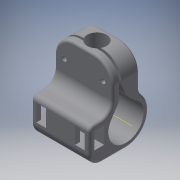
# Autodesk Inventor part: my_Sliding_Block_Complete
Saved by Autodesk Inventor 2016 (Build 200138000, 138)
## iProperties
Created: 2015-07-08
Part Number: my_Sliding_Block_Complete
Material: Generic
Document SubType Name: Modeling
Designer: Mathias L. Kjeldgaard
Density: 1 g/cm^3
Appearance: Default
Author: Mathias L. Kjeldgaard
Autodesk Inventor part; units mm, degrees
ref_plane "YZ Plane" through (0, 0, 0) normal (1, 0, 0) x (0, 1, 0)
sketch "Sketch1" plane through (0, 0, 0) normal (1, 0, 0) x (0, 1, 0)
  circle A0 centre (6.9957, 0) radius 7.5 construction
  circle A1 centre (6.9957, 0) radius 7.3
  line L0 (6.9957, -9.3) -> (-3.0043, -9.3)
  arc A2 (6.9957, -9.3) -> (13.8244, 6.3134) centre (6.9957, 0) ccw
  arc A3 (-8.0043, -4.3) -> (-3.0043, -9.3) centre (-3.0043, -4.3) ccw
  line L1 (6.9957, 0) -> (6.9957, 23.3) construction
  line L2 (12.4957, 4.8) -> (12.4957, 5.099)
  line L3 (12.4957, 9.7077) -> (12.4957, 23.3)
  arc A4 (12.4957, 9.7077) -> (13.8244, 6.3134) centre (17.4957, 9.7077) ccw
  line L4 (12.4957, 23.3) -> (5.0957, 23.3)
  line L5 (6.9957, 9.3) -> (5.0957, 9.3) construction
  line L6 (5.0957, 23.3) -> (5.0957, 16.4842)
  line L7 (12.4957, 9.7077) -> (12.4957, 4.8) construction
  line L8 (11.4281, 5.9069) -> (10.4435, 6.4345)
  arc A5 (5.0957, 16.4842) -> (11.4281, 5.9069) centre (17.0957, 16.4842) ccw
  line L9 (4.0957, 23.3) -> (1.4957, 23.3)
  line L10 (4.0957, 23.3) -> (4.0957, 10.3433)
  line L11 (1.4957, 23.3) -> (1.4957, 10.5)
  line L12 (-8.0043, 3.5) -> (-8.0043, -3.5)
  line L13 (-8.0043, -3.5) -> (-8.0043, -4.3)
  line L14 (-8.0043, 3.5) -> (-8.0043, 3.5)
  line L15 (-6.0043, 5.5) -> (-3.5043, 5.5)
  arc A6 (-3.5043, 5.5) -> (1.4957, 10.5) centre (-3.5043, 10.5) ccw
  line L16 (3.2629, 7.5803) -> (0.9116, 4.0341)
  arc A7 (3.2629, 7.5803) -> (4.0957, 10.3433) centre (-0.9043, 10.3433) ccw
  arc A8 (-6.0043, 5.5) -> (-8.0043, 3.5) centre (-6.0043, 3.5) ccw
  point P0 (0, 0)
  point P1 (12.4957, 7.4993)
  point P2 (6.9957, 7.3)
  point P3 (4.0957, 8.8363)
  point P4 (-8.0043, 5.5)
  dimension "d0" = 0.2
  dimension "d2" = 2
  dimension "d4" = 5
  dimension "d8" = 5
  dimension "d9" = 11
  dimension "d11" = 14
  dimension "d12" = 3.8
  dimension "d18" = 12
  dimension "d29" = 11
  dimension "d30" = 1
  dimension "d31" = 0
  dimension "d36" = 7
  dimension "d38" = 2
  dimension "d39" = 5
  dimension "d40" = 5
  dimension "d41" = 2
  dimension "d42" = 15
  dimension "d44" = 13
  constraints: 34 end point, 20 point on circle, 17 tangent, 11 point on line, 8 centre point, 6 perpendicular, 3 coincident, 3 parallel, 2 collinear, 1 horizontal, 2 other
  measures "d2" radial gap between concentric circles of A2 A1
  measures "d4" radius of A3
  measures "d8" radius of A4
  measures "d9" diameter of L3 L1
  measures "d11" distance from line of L5.start L4
  measures "d12" diameter of L6 L1
  measures "d18" radius of A5
  measures "d29" diameter of L11 L1
  measures "d30" distance between parallel lines of L6 L10
  measures "d31" distance from line of L1.end L9
  measures "d36" distance of L12.start L12.end
  measures "d38" distance of L12.start point (-8.004, 5.5)
  measures "d39" radius of A6
  measures "d40" radius of A7
  measures "d41" radius of A8
  measures "d42" distance from line of point (6.996, 0) L12
  measures "d44" horizontal distance of point (6.996, 0) A8.centre
ref_plane "Work Plane1" through (9.8693, -0.2503, -7.246) normal (1, 0, 0) x (0, 1, 0)
ref_plane "Work Plane2" through (-14.1307, -0.2503, -7.246) normal (-1, 0, 0) x (0, 0, 1)
extrude "Main body" add sketch "Sketch1" against normal up to surface (24 mm away) from surface at 9.8693 contours A1 L8 A5 L6 L4 L3 A4 A2 L0 A3 L13 L12 A8 L15 A6 L11 L9 L10 A7 L16
sketch "Sketch3" plane through (-14.1307, 5.0957, 23.3) normal (0, 0, 1) x (1, 0, 0)
  line L0 (24, 9.146) -> (24, -5.346) construction
  line L1 (0, -4.45) -> (0, 8.25) construction
  line L2 (0, -5.346) -> (0, 9.146) construction
  line L3 (0, 1.9) -> (24, 1.9) construction
  circle A0 centre (12, 1.9) radius 4
  point P0 (14.1307, -5.0957)
  dimension "d26" = 8
  constraints: 3 midpoint, 2 end point, 1 centre point
  measures "d26" diameter of A0
extrude "8mm hul" cut sketch "Sketch3" against normal blind 18.25
sketch "Sketch4" plane through (-14.1307, 1.4957, 10.5) normal (0, -1, 0) x (1, 0, 0)
  line L0 (0, 12.8) -> (0, 0) construction
  line L1 (0, 0) -> (24, 0) construction
  line L2 (24, 0) -> (24, 12.8) construction
  line L3 (0, 12.8) -> (24, 12.8) construction
  line L4 (8, 12.8) -> (16, 12.8) construction
  line L5 (9.245, 12.8) -> (14.755, 12.8) construction
  line L6 (8.4801, 12.8) -> (8.4801, 0) construction
  line L7 (15.5199, 12.8) -> (15.5199, 0) construction
  line L8 (15.5199, 12.8) -> (8.4801, 0) construction
  line L9 (12, 6.4) -> (12, 12.8) construction
  line L10 (8, 12.8) -> (8, 0) construction
  line L11 (16, 12.8) -> (16, 0) construction
  circle A0 centre (4, 5) radius 1
  circle A1 centre (20, 5) radius 1
  line L12 (20, 5) -> (4, 5) construction
  point P0 (14.1307, -10.5)
  dimension "d45" = 4
  dimension "d46" = 4
  dimension "d47" = 2
  dimension "d48" = 2
  dimension "d49" = 4
  dimension "d50" = 4
  dimension "d51" = 4
  dimension "d54" = 5
  constraints: 14 end point, 4 perpendicular, 4 point on line, 2 centre point, 2 midpoint, 1 parallel, 3 other
  measures "d45" distance between parallel lines of L9 L10
  measures "d46" distance between parallel lines of L11 L9
  measures "d47" diameter of A0
  measures "d48" diameter of A1
  measures "d49" distance from line of L2 L12.start
  measures "d50" distance from line of L0 L12.end
  measures "d51" distance from line of L11 L12.start
  measures "d54" distance between parallel lines of L1 L12
extrude "4mm Fastspændingshuller" cut sketch "Sketch4" against normal blind 10.25
sketch "Sketch5" plane through (-14.1307, 1.4957, 10.5) normal (0, -1, 0) x (1, 0, 0)
  line L0 (0, 12.8) -> (0, 0) construction
  line L1 (24, 0) -> (24, 12.8) construction
  line L2 (0, 12.8) -> (24, 12.8) construction
  line L3 (0, 4.8) -> (0, 0)
  line L4 (24, 0) -> (24, 4.8)
  line L5 (16, 12.8) -> (8, 12.8)
  arc A0 (8, 12.8) -> (0, 4.8) centre (8, 4.8) ccw
  arc A1 (24, 4.8) -> (16, 12.8) centre (16, 4.8) ccw
  line L6 (24, 0) -> (24, 4.8)
  line L7 (8, 12.8) -> (0, 12.8)
  line L8 (0, 12.8) -> (0, 4.8)
  line L9 (24, 12.8) -> (24, 4.8)
  line L10 (24, 12.8) -> (16, 12.8)
  point P0 (14.1307, -10.5)
  dimension "d57" = 8
  constraints: 16 end point, 7 tangent, 6 collinear, 5 point on circle, 5 point on line, 2 centre point, 1 equal radius, 1 perpendicular
  measures "d57" radius of A0
extrude "Afrunding v/ 8mm stang" cut sketch "Sketch5" against normal up to surface (11 mm away)
sketch "Sketch6" plane through (-14.1307, -3.0043, -9.3) normal (-1, 0, 0) x (0, 0, 1)
  arc A0 (15.6134, 16.8287) -> (0, 10) centre (9.3, 10) ccw construction
  line L0 (5.8, 1) -> (12.8, 1)
  line L1 (12.8, 1) -> (12.8, -3)
  line L2 (12.8, -3) -> (5.8, -3)
  line L3 (5.8, -3) -> (5.8, 1)
  point P0 (9.3, 3.0043)
  dimension "d60" = 7
  dimension "d61" = 4
  dimension "d62" = 9
  dimension "d63" = 3.5
  dimension "d64" = 3.5
  constraints: 8 end point, 2 parallel, 1 horizontal, 1 perpendicular
  measures "d60" distance between parallel lines of L3 L1
  measures "d61" distance between parallel lines of L0 L2
  measures "d62" distance from line of A0.centre L0
  measures "d63" distance from line of A0.centre L1
  measures "d64" distance from line of A0.centre L3
extrude "GT2 Belte hul Stort" cut sketch "Sketch6" against normal up to surface (24 mm away)
sketch "Sketch7" plane through (-14.1307, -8.0043, -4.3) normal (0, -1, 0) x (1, 0, 0)
  line L0 (0, 7.8) -> (0, 0) construction
  line L1 (24, 0.8) -> (24, 7.8) construction
  line L2 (0, 0.8) -> (24, 0.8) construction
  line L3 (0, 7.8) -> (0, 0.8) construction
  line L4 (0, 7.8) -> (24, 7.8) construction
  line L5 (2, 7.8) -> (6, 7.8)
  line L6 (6, 7.8) -> (6, 0.8)
  line L7 (6, 0.8) -> (2, 0.8)
  line L8 (2, 0.8) -> (2, 7.8)
  line L9 (18, 7.8) -> (22, 7.8)
  line L10 (22, 7.8) -> (22, 0.8)
  line L11 (22, 0.8) -> (18, 0.8)
  line L12 (18, 0.8) -> (18, 7.8)
  point P0 (14.1307, 4.3)
  dimension "d67" = 2
  dimension "d68" = 4
  dimension "d69" = 2
  dimension "d70" = 4
  constraints: 16 end point, 4 parallel, 4 point on line, 2 horizontal, 2 perpendicular
  measures "d67" distance between parallel lines of L8 L0
  measures "d68" distance between parallel lines of L6 L8
  measures "d69" distance between parallel lines of L1 L10
  measures "d70" distance between parallel lines of L12 L10
extrude "GT2 belte hul Lille" cut sketch "Sketch7" against normal blind 4.25
fillet "Ydre fillet" radius 1 16 edges at (9.8693, 1.9957, -9.3) (9.8693, -6.5398, -7.8355) (9.8693, -8.0043, -0.4) (9.8693, -7.4185, 4.9142) (9.8693, -4.7543, 5.5) (9.8693, 0.0313, 6.9645) (9.8693, 1.4957, 12.9) (7.5262, 1.4957, 20.9569) (-2.1307, 1.4957, 23.3) (-11.7875, 1.4957, 20.9569) (9.8693, 15.5164, -3.7266) (9.8693, 12.8397, 7.8852) (9.8693, 12.4957, 12.5039) (-11.7875, 12.4957, 20.9569) (-2.1307, 12.4957, 23.3) (7.5262, 12.4957, 20.9569)
equation "\"d29\" = d9"
equation "\"d46\" = d45"
equation "\"d48\" = d47"
equation "\"d49\" = d51"
equation "\"d50\" = d49"
equation "\"d63\" = d64"
equation "\"d69\" = d67"
equation "\"d70\" = d68"
equation "\"d10\" = d9"
body "Solid1"
